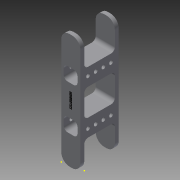
# Autodesk Inventor part: 150mm Link
Saved by Autodesk Inventor 2015 (Build 190159000, 159)
## iProperties
Created: 2016-11-30
Part Number: 150mm Link
Material: Generic
Document SubType Name: Modeling
Designer: Rudge-Top
Density: 1 g/cm^3
Appearance: Default
Author: Rudge-Top
Autodesk Inventor part; units mm, degrees
ref_plane "YZ Plane" through (0, 0, 0) normal (1, 0, 0) x (0, 1, 0)
ref_plane "XZ Plane" through (0, 0, 0) normal (0, 1, 0) x (-1, 0, 0)
ref_plane "XY Plane" through (0, 0, 0) normal (0, 0, 1) x (1, 0, 0)
sketch "Sketch1" plane through (0, 0, 0) normal (1, 0, 0) x (0, 1, 0)
  line L0 (120, 0) -> (150, 0)
  line L1 (150, 0) -> (150, -40)
  line L2 (150, -40) -> (120, -40)
  line L3 (150, 5) -> (0, 5)
  line L4 (0, -45) -> (150, -45)
  line L5 (150, 0) -> (150, 5)
  line L6 (150, -40) -> (150, -45)
  line L7 (0, -40) -> (0, -45)
  line L8 (0, 0) -> (0, 5)
  line L9 (115, -5) -> (115, -35)
  arc A0 (120, 0) -> (115, -5) centre (120, -5) ccw
  arc A1 (115, -35) -> (120, -40) centre (120, -35) ccw
  line L10 (87.5, 0) -> (62.5, 0)
  line L11 (57.5, -5) -> (57.5, -35)
  line L12 (62.5, -40) -> (87.5, -40)
  line L13 (92.5, -35) -> (92.5, -5)
  arc A2 (87.5, -40) -> (92.5, -35) centre (87.5, -35) ccw
  arc A3 (57.5, -35) -> (62.5, -40) centre (62.5, -35) ccw
  arc A4 (62.5, 0) -> (57.5, -5) centre (62.5, -5) ccw
  arc A5 (92.5, -5) -> (87.5, 0) centre (87.5, -5) ccw
  line L14 (0, 0) -> (30, 0)
  line L15 (35, -5) -> (35, -35)
  line L16 (30, -40) -> (0, -40)
  arc A6 (35, -5) -> (30, 0) centre (30, -5) ccw
  arc A7 (30, -40) -> (35, -35) centre (30, -35) ccw
  point P0 (57.5, -40)
  point P1 (92.5, -40)
  point P2 (35, 0)
  dimension "d1" = 150
  dimension "d2" = 40
  dimension "d3" = 90
  dimension "d4" = 5
  dimension "d5" = 35
  dimension "d6" = 5
  dimension "d7" = 35
  dimension "d8" = 5
  dimension "d9" = 22.5
  dimension "d10" = 5
  dimension "d11" = 35
  dimension "d12" = 5
  constraints: 34 end point, 16 point on circle, 16 tangent, 9 point on line, 8 centre point, 8 perpendicular, 5 equal radius, 3 horizontal, 2 parallel
  measures "d1" distance of L8.start L0.end
  measures "d2" distance of L0.end L1.end
  measures "d3" angle of L0 L1
  measures "d4" distance between parallel lines of L0 L3
  measures "d5" distance between parallel lines of L1 L9
  measures "d6" radius of A0
  measures "d7" distance of point (92.5, -40) point (57.5, -40)
  measures "d8" distance between parallel lines of L3 L10
  measures "d9" distance between parallel lines of L13 L9
  measures "d10" radius of A2
  measures "d11" distance of L8.start point (35, 0)
  measures "d12" radius of A6
extrude "Extrusion1" add sketch "Sketch1" along normal blind 25 contours A0 L9 A1 L2 L6 L4 L7 L16 A7 L15 A6 L14 L8 L3 L5 L0
sketch "Sketch2" plane through (25, 0, 0) normal (1, 0, 0) x (0, 0, -1)
  arc A0 (35, 57.5) -> (40, 62.5) centre (35, 62.5) ccw projected
  line L0 (35, 57.5) -> (5, 57.5) projected
  arc A1 (0, 62.5) -> (5, 57.5) centre (5, 62.5) ccw projected
  line L1 (0, 62.5) -> (0, 87.5) projected
  arc A2 (5, 92.5) -> (0, 87.5) centre (5, 87.5) ccw projected
  line L2 (5, 92.5) -> (35, 92.5) projected
  arc A3 (40, 87.5) -> (35, 92.5) centre (35, 87.5) ccw projected
  line L3 (40, 87.5) -> (40, 62.5) projected
  line L4 (0, 0) -> (0, 30) projected
  arc A4 (5, 35) -> (0, 30) centre (5, 30) ccw projected
  line L5 (5, 35) -> (35, 35) projected
  arc A5 (40, 30) -> (35, 35) centre (35, 30) ccw projected
  line L6 (40, 30) -> (40, 0) projected
  line L7 (40, 0) -> (45, 0) projected
  line L8 (45, 0) -> (45, 150) projected
  line L9 (45, 150) -> (40, 150) projected
  line L10 (40, 150) -> (40, 120) projected
  arc A6 (35, 115) -> (40, 120) centre (35, 120) ccw projected
  line L11 (35, 115) -> (5, 115) projected
  arc A7 (0, 120) -> (5, 115) centre (5, 120) ccw projected
  line L12 (0, 120) -> (0, 150) projected
  line L13 (0, 150) -> (-5, 150) projected
  line L14 (-5, 150) -> (-5, 0) projected
  line L15 (-5, 0) -> (0, 0) projected
  circle A8 centre (35, 45.25) radius 2.5
  circle A9 centre (25, 45.25) radius 2.5
  circle A10 centre (15, 45.25) radius 2.5
  circle A11 centre (5, 45.25) radius 2.5
  circle A12 centre (35, 104.75) radius 2.5
  circle A13 centre (25, 104.75) radius 2.5
  circle A14 centre (15, 104.75) radius 2.5
  circle A15 centre (5, 104.75) radius 2.5
  dimension "d15" = 5
  dimension "d16" = 5
  dimension "d17" = 5
  dimension "d18" = 5
  dimension "d19" = 10
  dimension "d20" = 20
  dimension "d21" = 30
  dimension "d22" = 40
  dimension "d23" = 5
  dimension "d24" = 5
  dimension "d25" = 5
  dimension "d26" = 5
  dimension "d27" = 12.25
  dimension "d28" = 12.25
  dimension "d29" = 12.25
  dimension "d30" = 12.25
  dimension "d31" = 12.25
  dimension "d32" = 12.25
  dimension "d33" = 12.25
  dimension "d34" = 12.25
  constraints: 8 centre point
  measures "d15" diameter of A8
  measures "d16" diameter of A9
  measures "d17" diameter of A10
  measures "d18" diameter of A11
  measures "d19" distance from line of L14 A11.centre
  measures "d20" distance from line of A10.centre L14
  measures "d21" distance from line of A9.centre L14
  measures "d22" distance from line of A8.centre L14
  measures "d23" diameter of A12
  measures "d24" diameter of A13
  measures "d25" diameter of A14
  measures "d26" diameter of A15
  measures "d27" distance from line of A12.centre L2
  measures "d28" distance from line of L2 A13.centre
  measures "d29" distance from line of L2 A14.centre
  measures "d30" distance from line of L2 A15.centre
  measures "d31" distance from line of A8.centre L0
  measures "d32" distance from line of A9.centre L0
  measures "d33" distance from line of A10.centre L0
  measures "d34" distance from line of A11.centre L0
extrude "Extrusion2" cut sketch "Sketch2" against normal blind 25 contours A8 | A9 | A10 | A11 | A12 | A13 | A14 | A15
fillet "Fillet1" radius 11 8 edges at (25, 0, 2.5) (0, 0, 2.5) (25, 0, -42.5) (0, 0, -42.5) (25, 150, 2.5) (25, 150, -42.5) (0, 150, -42.5) (0, 150, 2.5)
sketch "Sketch3" plane through (0, 11, -45) normal (0, 0, -1) x (-1, 0, 0)
  line L0 (0, 51.5) -> (-25, 51.5) projected
  arc A0 (0, 128) -> (-11, 139) centre (-11, 128) ccw projected
  line L1 (-11, 139) -> (-14, 139) projected
  arc A1 (-14, 139) -> (-25, 128) centre (-14, 128) ccw projected
  line L2 (-25, 0) -> (-25, 128) projected
  arc A2 (-25, 0) -> (-14, -11) centre (-14, 0) ccw projected
  line L3 (-11, -11) -> (-14, -11) projected
  arc A3 (-11, -11) -> (0, 0) centre (-11, 0) ccw projected
  line L4 (0, 0) -> (0, 128) projected
  line L5 (-25, 51.5) -> (-25, 46.5) projected
  line L6 (-25, 46.5) -> (-25, 51.5) projected
  line L7 (-25, 51.5) -> (-25, 76.5) projected
  line L8 (-25, 76.5) -> (-25, 81.5) projected
  line L9 (-25, 81.5) -> (-25, 76.5) projected
  line L10 (-25, 76.5) -> (-25, 51.5) projected
  line L11 (-25, 91.25) -> (-25, 96.25) projected
  line L12 (-25, 91.25) -> (-25, 96.25) projected
  line L13 (-25, 31.75) -> (-25, 36.75) projected
  line L14 (-25, 31.75) -> (-25, 36.75) projected
  line L15 (-25, 31.75) -> (-25, 36.75) projected
  line L16 (-25, 31.75) -> (-25, 36.75) projected
  line L17 (-25, 91.25) -> (-25, 96.25) projected
  line L18 (-25, 91.25) -> (-25, 96.25) projected
  line L19 (-25, 128) -> (-25, 109) projected
  line L20 (-25, 109) -> (-25, 104) projected
  line L21 (-25, 104) -> (-25, 109) projected
  line L22 (-25, 109) -> (-25, 128) projected
  line L23 (-25, 128) -> (-25, 0) projected
  line L24 (-25, 0) -> (-25, 19) projected
  line L25 (-25, 19) -> (-25, 24) projected
  line L26 (-25, 24) -> (-25, 19) projected
  line L27 (-25, 19) -> (-25, 0) projected
  line L28 (-25, 0) -> (-25, 128) projected
  line L29 (-8.2218, 26.5) -> (-16.2218, 26.5)
  line L30 (-21.2218, 31.5) -> (-21.2218, 39)
  line L31 (-16.2218, 44) -> (-8.2218, 44)
  line L32 (-3.2218, 39) -> (-3.2218, 31.5)
  arc A4 (-21.2218, 31.5) -> (-16.2218, 26.5) centre (-16.2218, 31.5) ccw
  arc A5 (-16.2218, 44) -> (-21.2218, 39) centre (-16.2218, 39) ccw
  arc A6 (-3.2218, 39) -> (-8.2218, 44) centre (-8.2218, 39) ccw
  arc A7 (-8.2218, 26.5) -> (-3.2218, 31.5) centre (-8.2218, 31.5) ccw
  line L33 (-8.2218, 84) -> (-16.2218, 84)
  line L34 (-21.2218, 89) -> (-21.2218, 96.5)
  line L35 (-16.2218, 101.5) -> (-8.2218, 101.5)
  line L36 (-3.2218, 96.5) -> (-3.2218, 89)
  arc A8 (-21.2218, 89) -> (-16.2218, 84) centre (-16.2218, 89) ccw
  arc A9 (-16.2218, 101.5) -> (-21.2218, 96.5) centre (-16.2218, 96.5) ccw
  arc A10 (-3.2218, 96.5) -> (-8.2218, 101.5) centre (-8.2218, 96.5) ccw
  arc A11 (-8.2218, 84) -> (-3.2218, 89) centre (-8.2218, 89) ccw
  point P0 (0, -11)
  point P1 (-21.2218, 44)
  point P2 (-21.2218, 26.5)
  point P3 (-3.2218, 44)
  dimension "d38" = 18
  dimension "d39" = 17.5
  dimension "d40" = 55
  dimension "d41" = 5
  dimension "d42" = 5
  dimension "d43" = 55
  constraints: 16 end point, 16 point on circle, 16 tangent, 8 centre point, 6 equal radius, 6 point on line, 4 parallel, 2 horizontal, 2 perpendicular
  measures "d38" distance of point (-21.222, 44) point (-3.222, 44)
  measures "d39" distance of point (-21.222, 26.5) point (-21.222, 44)
  measures "d40" distance between parallel lines of L3 L31
  measures "d41" radius of A4
  measures "d42" radius of A8
  measures "d43" distance between parallel lines of L1 L33
extrude "Extrusion3" cut sketch "Sketch3" against normal blind 100 contours L29 A4 L30 A5 L31 A6 L32 A7 | L33 A8 L34 A9 L35 A10 L36 A11
sketch "Sketch4" plane through (0, 11, 5) normal (0, 0, 1) x (1, 0, 0)
  line L0 (13.7515, 74.4502) -> (13.7515, 54.5408) construction
  line L1 (13.7515, 54.5408) -> (10.1902, 54.5408) construction
  line L2 (10.1902, 54.5408) -> (10.1902, 74.4502) construction
  line L3 (10.1902, 74.4502) -> (13.7515, 74.4502) construction
  point P0 (0, -11)
  constraints: 2 other
sketch "Sketch5" plane through (25, 0, 0) normal (1, 0, 0) x (0, 0, -1)
  point P0 (0, 0)
body "Solid1"
